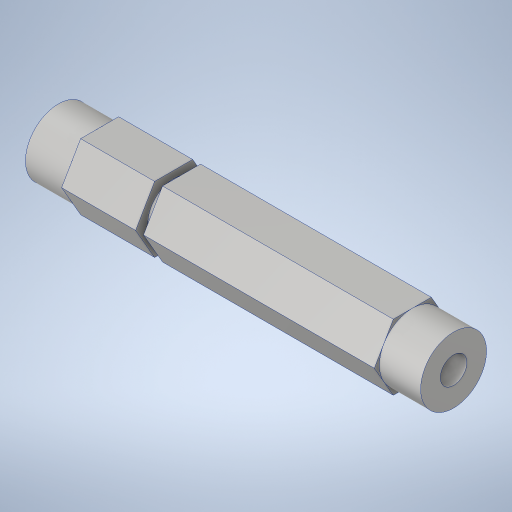
# Autodesk Inventor part: EL2-GB-005E-grove
Saved by Autodesk Inventor 2023.4 (Build 274418000, 418)
## iProperties
Created: 2025-01-18
Part Number: EL2-GB-005E-grove
Material: Aluminum 6061
Document SubType Name: Modeling
Designer: mavericks
Density: 2.7 g/cm^3
Appearance: Aluminum - Flat
Author: mavericks
Autodesk Inventor part; units mm, degrees
ref_plane "YZ Plane" through (0, 0, 0) normal (1, 0, 0) x (0, 1, 0)
ref_plane "XZ Plane" through (0, 0, 0) normal (0, 1, 0) x (-1, 0, 0)
ref_plane "XY Plane" through (0, 0, 0) normal (0, 0, 1) x (1, 0, 0)
sketch "Sketch1" plane through (0, 0, 0) normal (1, 0, 0) x (0, 1, 0)
  line L0 (0, -7.3323) -> (-6.35, -3.6662)
  line L1 (-6.35, -3.6662) -> (-6.35, 3.6662)
  line L2 (-6.35, 3.6662) -> (0, 7.3323)
  line L3 (0, 7.3323) -> (6.35, 3.6662)
  line L4 (6.35, 3.6662) -> (6.35, -3.6662)
  line L5 (6.35, -3.6662) -> (0, -7.3323)
  point P0 (0, 0)
  point P1 (0, 0)
  dimension "d0" = 12.7
  constraints: 12 end point, 1 coincident, 1 vertical, 13 other
  measures "d0" distance between parallel lines of L1 L4
extrude "Extrusion1" add sketch "Sketch1" along normal mid plane 60.2996
sketch "Sketch2" plane through (-30.1498, 0, 0) normal (-1, 0, 0) x (0, 0, 1)
  circle A0 centre (0, 0) radius 6.35
  dimension "d3" = 12.7
  constraints: 1 centre point, 1 coincident
  measures "d3" diameter of A0
extrude "Extrusion2" add sketch "Sketch2" along normal blind 7.9502
sketch "Sketch3" plane through (30.1498, 0, 0) normal (1, 0, 0) x (0, 0, -1)
  circle A0 centre (0, 0) radius 6.35
  line L0 (3.6662, 6.35) -> (-3.6662, 6.35) projected
  line L1 (-3.6662, 6.35) -> (-7.3323, 0) projected
  line L2 (-7.3323, 0) -> (-3.6662, -6.35) projected
  line L3 (-3.6662, -6.35) -> (3.6662, -6.35) projected
  line L4 (3.6662, -6.35) -> (7.3323, 0) projected
  line L5 (7.3323, 0) -> (3.6662, 6.35) projected
  dimension "d6" = 12.7
  constraints: 1 centre point, 1 coincident
  measures "d6" diameter of A0
extrude "Extrusion3" add sketch "Sketch3" along normal blind 7.9502 contours A0
sketch "Sketch4" plane through (38.1, 0, 0) normal (1, 0, 0) x (0, 0, -1)
  point P0 (0, 0)
  point P1 (0, 0)
  constraints: 1 coincident
hole "Hole1" at (38.1, 0, 0) direction (-1, 0, 0) diameter 5.1054 end through all clearance for "Flat Head Machine Screw (82)" size "#10" standard "Ansi Unified Screw Threads"
sketch "Sketch6" plane through (0, 0, 0) normal (0, 1, 0) x (-1, 0, 0)
  line L0 (30.1498, 6.35) -> (38.1, 6.35) projected
  line L1 (38.1, 6.35) -> (38.1, 2.5527) projected
  line L2 (38.1, 2.5527) -> (-38.1, 2.5527) projected
  line L3 (-38.1, 2.5527) -> (-38.1, 6.35) projected
  line L4 (-38.1, 6.35) -> (-30.1498, 6.35) projected
  line L5 (-30.1498, 6.35) -> (-30.1498, 7.3323) projected
  line L6 (-30.1498, 7.3323) -> (30.1498, 7.3323) projected
  line L7 (30.1498, 7.3323) -> (30.1498, 6.35) projected
  line L8 (38.1, -6.35) -> (30.1498, -6.35) projected
  line L9 (30.1498, -6.35) -> (30.1498, -7.3323) projected
  line L10 (30.1498, -7.3323) -> (-30.1498, -7.3323) projected
  line L11 (-30.1498, -7.3323) -> (-30.1498, -6.35) projected
  line L12 (-30.1498, -6.35) -> (-38.1, -6.35) projected
  line L13 (-38.1, -6.35) -> (-38.1, -2.5527) projected
  line L14 (-38.1, -2.5527) -> (38.1, -2.5527) projected
  line L15 (38.1, -2.5527) -> (38.1, -6.35) projected
  line L16 (38.1, 2.5527) -> (38.1, -2.5527) projected
  line L17 (38.1, 0) -> (-38.1, 0)
  line L18 (-38.1, 6.35) -> (-38.1, -6.35) projected
  line L19 (15.875, -7.3323) -> (14.351, -7.3323)
  line L20 (14.351, -7.3323) -> (14.351, -4.9784)
  line L21 (14.351, -4.9784) -> (15.875, -4.9784)
  line L22 (15.875, -4.9784) -> (15.875, -7.3323)
  point P0 (0, 0)
  dimension "d16" = 9.9568
  dimension "d17" = 1.524
  dimension "d18" = 22.225
  constraints: 10 end point, 2 midpoint, 2 parallel, 1 horizontal, 1 perpendicular, 1 point on line
  measures "d16" diameter of L21 L17
  measures "d17" distance of L20.end L21.end
  measures "d18" distance between parallel lines of L15 L22
revolve "Revolution1" cut sketch "Sketch6" angle 360 about axis through (-38.1, 0, 0) along (1, 0, 0) contours L10 L20 L21 L22
body "Solid1"
